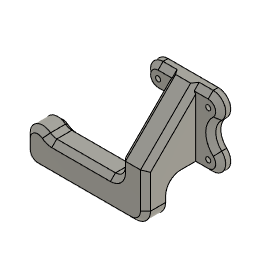
ChainsawHolderV2 v4 (Autodesk Fusion 360 design; units mm, degrees)
Autodesk Fusion 360 part; units mm, degrees
sketch "Sketch1" plane through (0, 0, 0) normal (0, 1, 0) x (1, 0, 0)
  circle A0 centre (0, 0) radius 17 construction
  line L0 (32, -17) -> (32, 83) construction
  line L1 (32, 83) -> (-50, 83) construction
  line L2 (-50, 83) -> (-50, -17) construction
  line L3 (59.6348, -53) -> (59.6348, 47)
  line L4 (59.6348, 47) -> (34.6348, 47)
  line L5 (34.6348, 47) -> (34.6348, -53)
  line L6 (59.6348, 47) -> (-60.3652, 47)
  line L7 (-60.3652, 47) -> (-60.3652, 17)
  line L8 (-60.3652, 17) -> (59.6348, 17)
  line L9 (59.6348, 17) -> (59.6348, 47)
  line L10 (34.6348, -53) -> (59.6348, -53)
  line L11 (-50, -17) -> (32, -17) construction
  line L12 (34.6348, -53) -> (9.6348, -53)
  line L13 (9.6348, -53) -> (9.6348, -28)
  line L14 (9.6348, -28) -> (34.6348, -28)
  line L15 (59.6348, -53) -> (84.6348, -53)
  line L16 (84.6348, -53) -> (84.6348, 17)
  line L17 (84.6348, 17) -> (59.6348, 17)
  circle A1 centre (22.1348, -40.5) radius 2.5
  circle A2 centre (72.1348, -40.5) radius 2.5
  circle A3 centre (72.1348, 4.5) radius 2.5
  circle A4 centre (22.1348, -40.5) radius 12.5
  circle A5 centre (72.1348, -40.5) radius 12.5
  circle A6 centre (72.1348, 4.5) radius 12.5
  arc A7 (80.5738, -4.7213) -> (80.5738, -31.2787) centre (92.726, -18) ccw
  circle A8 centre (-47.9373, 24.5) radius 12.428
  circle A9 centre (45.2444, 32.6096) radius 14.3904
  circle A10 centre (-47.8652, 34.5) radius 12.5
  dimension "d1" = 34
  dimension "d3" = 32
  dimension "d10" = 100
  dimension "d11" = 120
  dimension "d12" = 30
  dimension "d45" = 25
  dimension "d46" = 25
  dimension "d47" = 25
  dimension "d48" = 25
  dimension "d49" = 70
  dimension "d50" = 5
  dimension "d51" = 12.5
  dimension "d52" = 12.5
  dimension "d53" = 5
  dimension "d54" = 5
  dimension "d55" = 12.5
  dimension "d56" = 12.5
  dimension "d57" = 12.5
  dimension "d58" = 12.5
  dimension "d66" = 18
  dimension "d76" = 25
  dimension "d77" = 7.5
  constraint coincident A0.centre origin
  constraint vertical L0
  constraint horizontal L1
  constraint vertical L2
  constraint vertical L3
  constraint horizontal L4
  constraint vertical L5
  constraint horizontal L6
  constraint vertical L7
  constraint horizontal L8
  constraint vertical L9
  constraint tangent A0 L8
  constraint perpendicular L3 L10
  constraint perpendicular L2 L11
  constraint tangent A0 L11
  constraint perpendicular L5 L12
  constraint perpendicular L10 L13
  constraint coincident L5 L14.end
  constraint perpendicular L5 L14
  constraint perpendicular L3 L15
  constraint perpendicular L10 L16
  constraint coincident L3 L8.end
  constraint perpendicular L3 L17
  constraint concentric A1 A4
  constraint tangent L12 A4
  constraint concentric A2 A5
  constraint tangent L15 A5
  constraint concentric A3 A6
  constraint tangent L16 A6
  constraint tangent A6 A7
  constraint coincident A6 A7.start
  constraint coincident A5 A7.end
  constraint tangent A5 A7
  constraint tangent L9 A9
  constraint tangent L4 A9
  constraint tangent L6 A10
  constraint tangent L7 A10
  constraint tangent L7 A8
  measures "d1" diameter of A0
  measures "d3" distance of A0.centre L0
  measures "d10" distance of L5.end L4.end
  measures "d11" distance of L3.end L6.end
  measures "d12" distance of L3.end L8.end
  measures "d45" distance of L3 L5
  measures "d46" distance of L3.start L15.end
  measures "d47" distance of L5.end L12.end
  measures "d48" distance of L12.end L13.end
  measures "d49" distance of L15.end L16.end
  measures "d50" diameter of A1
  measures "d51" distance of L12 A1.centre
  measures "d52" distance of L13 A1.centre
  measures "d53" diameter of A2
  measures "d54" diameter of A3
  measures "d55" distance of L15 A2.centre
  measures "d56" distance of L17 A3.centre
  measures "d57" distance of L16 A3.centre
  measures "d58" distance of L16 A2.centre
  measures "d66" radius of A7
  measures "d76" diameter of A10
  measures "d77" distance of L8 A8.centre
extrude "Extrude4" add sketch "Sketch1" along normal blind 10 contours L3 L17 A6 | L3 L5 L8 L10 | L3 A5 A6 A7 | A6 | L3 L15 A5 | A5 | L5 L14 A4 | A4 | L5 L12 A4
extrude "Extrude5" add sketch "Sketch1" against normal blind 25 contours L3 L5 L8 L10
extrude "Extrude6" add sketch "Sketch1" against normal blind 25 from surface at -25 contours L3 L5 L8 L9 A9 | L3 L5 L8 L10 | L5 A9 | L5 L6 L8 A8 A9 A10 | L4 L5 L6 A9 | L5 A9 | L8 A8 | L8 A8 A10 | A8 A10 | L7 A8 A10 | A8 A10
fillet "Fillet6" radius 10 1 edges at (34.6348, -37.5, -17)
fillet "Fillet6" radius 10 1 edges at (-38.0274, -37.5, -17)
fillet "Fillet7" radius 10 1 edges at (47.1348, -25, -17)
chamfer "Chamfer2" distance 50 angle 45 1 edges at (47.1348, -50, 53)
chamfer "Chamfer3" distance 5 angle 45 25 edges at (-4.6376, -50, -17) (31.7058, -50, -14.0711) (34.6348, -50, -2) (59.6348, -50, -14.8048) (55.4199, -50, -42.7852) (-1.3104, -50, -47) (-56.7041, -50, -43.3388) (-60.3652, -50, -29.5) (-53.3156, -50, -13.2961) (-37.2245, -50, -16.4347) (-4.6376, -25, -17) (-37.2245, -25, -16.4347) (-53.3156, -25, -13.2961) (-60.3652, -25, -29.5) (-56.7041, -25, -43.3388) (-1.3104, -25, -47) (55.4199, -25, -42.7852) (59.6348, -25, -29.8048) (59.6348, -22.0711, -19.9289) (59.6348, -7.5, -17) (31.7058, -25, -14.0711) (34.6348, -25, 28) (59.6348, -25, 28) (34.6348, -2.5, -17) (34.6348, -22.0711, -19.9289)
chamfer "Chamfer4" distance 5 angle 45 8 edges at (83.7863, 0, 45.0268) (74.726, 0, 18) (83.7863, 0, -9.0268) (63.3848, 0, -17) (63.3848, 0, 53) (30.8848, 0, 53) (9.6348, 0, 40.5) (28.3848, 0, 28)
equation "d3 = ( ( 34 / 2 ) * 1 mm ) + 15 mm"
equation "d51 = ( 25 / 2 ) * 1 mm"
equation "d52 = ( 25 / 2 ) * 1 mm"
equation "d55 = ( 25 / 2 ) * 1 mm"
equation "d56 = ( 25 / 2 ) * 1 mm"
equation "d57 = ( 25 / 2 ) * 1 mm"
equation "d58 = ( 25 / 2 ) * 1 mm"
